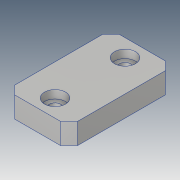
# Autodesk Inventor part: 200-50-WHEEL-CONNECTOR-30MM-02
Saved by Autodesk Inventor 2018.2 (Build 222227000, 227)
## iProperties
Manager: feesmrt
Company: FRANC0R
Created: 2017-12-05
Part Number: 200-50-WHEEL-CONNECTOR-30MM-02
Material: Aluminium 6061
Document SubType Name: Modeling
Designer: feesmrt
Density: 2.7 g/cm^3
Appearance: Aluminium - flach
Project: Rescue Robot
Cost Center: -
Engineer: feesmrt
Authority: feesmrt
Description: Wheel Connector 30mm Part 2
Stock Number: 200-50-WHEEL-CONNECTOR-30MM-02
Author: feesmrt
Subject: Rescue Robot
Title: Wheel Connector 30mm Part 2
Revision Number: 1
Autodesk Inventor part; units mm, degrees
ref_plane "YZ Plane" through (0, 0, 0) normal (1, 0, 0) x (0, 1, 0)
ref_plane "XZ Plane" through (0, 0, 0) normal (0, 1, 0) x (-1, 0, 0)
ref_plane "XY Plane" through (0, 0, 0) normal (0, 0, 1) x (1, 0, 0)
derived "200-50-WHEEL-CONNECTOR-30MM-01.ipt"
sketch "Skizze" plane through (15, -25, -30) normal (0, 0, -1) x (-1, 0, 0)
  circle A0 centre (15, 8.3) radius 2.5
  line L0 (30, 16.6) -> (0, 16.6)
  line L1 (0, 0) -> (0, 16.6)
  line L2 (0, 0) -> (30, 0)
  line L3 (30, 16.6) -> (30, 0)
  circle A1 centre (15, 41.7) radius 2.5
  line L4 (0, 33.4) -> (30, 33.4)
  line L5 (30, 50) -> (30, 33.4)
  line L6 (30, 50) -> (0, 50)
  line L7 (0, 33.4) -> (0, 50)
  line L8 (0, 16.6) -> (0, 24.6)
  line L9 (0, 24.6) -> (0, 25.4)
  line L10 (0, 25.4) -> (0, 33.4)
  line L11 (30, 33.4) -> (30, 25.4)
  line L12 (30, 25.4) -> (30, 24.6)
  line L13 (30, 24.6) -> (30, 16.6)
  point P0 (15, 25)
sketch "Skizze2" plane through (0, 0, 0) normal (0, 0, 1) x (1, 0, 0)
  line L0 (-15, 25) -> (15, 25)
  line L1 (15, 25) -> (15, -25)
  line L2 (15, -25) -> (-15, -25)
  line L3 (-15, -25) -> (-15, 25)
  point P0 (0, 0)
  constraints: 8 end point, 2 parallel, 1 horizontal, 1 perpendicular
extrude "Grundkörper" add sketch "Skizze2" along normal mid plane 10
sketch "Skizze3" plane through (0, 0, 5) normal (0, 0, 1) x (1, 0, 0)
  circle A0 centre (0, 16.7) radius 2.5 projected
  circle A1 centre (0, -16.7) radius 2.5 projected
  point P0 (0, 0)
hole "DIN7984_M5_Boh" at (0, 16.7, 5) at (0, -16.7, 5) direction (0, 0, -1) diameter 5.5 end through all counterbore diameter 10 counterbore depth 3.9
chamfer "Fase1" distance 4 angle 45 4 edges at (15, -25, 0) (15, 25, 0) (-15, 25, 0) (-15, -25, 0)
